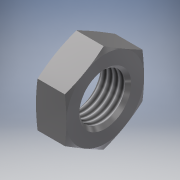
# Autodesk Inventor part: D-801
Saved by Autodesk Inventor 2016 SP2 (Build 200236200, 236)
## iProperties
Category: PARTsolutions
Company: BIMBA
Created: 2017-03-17
Part Number: D-801
Catalog Web Link: www.cadenas.de
Description: Jam Nut-Bimba Nut for Alignment Couplers
Vendor: BIMBA
Document SubType Name: Modeling
Designer: psAdmin
Manufacturer: BIMBA
Mass: 5.17328 g
Surface Area: 6.36956 cm^2
Volume: 0.659017 cm^3
Density: 7.85 g/cm^3
Material: Steel, Carbon
Appearance: Semi-Polished
PSOL_IDENT_0: {$CADENAS_DATA\23d-libs\bimba\bimba\bimba_imperial\bimba_full_line\related_products\ac_jam_nut.prj},
PSOL_IDENT_1: 156 {VTYP=3D},{NB=D-801},{LINA=D-801},{NN=Jam Nut},{DATE=01.09.2016 11:36:35},{GEOMDATE=06.09.2013 0
PSOL_IDENT_2: 7:06:46},{VERSION=},{LINEID=30},{LINESUBID=-1},{WBVAR=MAT}  {NB=D-801},{LINA=D-801},{KT=DUMMY},{PN=D
PSOL_IDENT_3: -801},{PN1=D-801},{SIZE=3/8-24},{MAT=},{J=0.22},{JJ=0.22000},{T=3/8-24},{TT=0.37500},{H=0.56},{HEX=0
PSOL_IDENT_4: .560},{COLOR=0.75,0.75,0.75,0.00}
NN: Jam Nut
NT: Bimba Nut for Alignment Couplers
NB: D-801
NBSYN: $PN.
LINA: D-801
PN: D-801
SIZE: 3/8-24 [D-801]
MAT: Zinc-Plated Carbon Steel
J: 0.22
T: 3/8-24
H: 0.56
SUPPLIER: BIMBA
ARTICLENO: D-801
BOMINFO: D-801
CREATOR: CADENAS GmbH
Title: D-801
Author: Cadenas PARTsolutions
Comments: Bimba Nut for Alignment Couplers
Autodesk Inventor part; units mm, degrees
sketch "Sketch_1" plane through (0, 0, 0) normal (0, 0, 1) x (1, 0, 0)
  line L0 (2.794, 0) -> (-2.794, 0)
  line L1 (-2.794, 4.7625) -> (-2.2212, 4.1897)
  line L2 (-2.2212, 4.1897) -> (2.2212, 4.1897)
  line L3 (2.2212, 4.1897) -> (2.794, 4.7625)
  line L4 (2.794, 4.7625) -> (2.794, 7.112)
  line L5 (2.794, 7.112) -> (2.4129, 8.5344)
  line L6 (2.4129, 8.5344) -> (-2.4129, 8.5344)
  line L7 (-2.4129, 8.5344) -> (-2.794, 7.112)
  line L8 (-2.794, 7.112) -> (-2.794, 4.7625)
  constraints: 18 end point
revolve "Revolution1" add sketch "Sketch_1" angle 360 about axis through (2.794, 0, 0) along (1, 0, 0)
thread "Thread1" size "3/8-24 UNF" class "2B" standard "ANSI Unified Screw Threads" full length
sketch "Sketch_2" plane through (0, 0, 0) normal (1, 0, 0) x (0, 1, 0)
  circle A0 centre (0, 0) radius 14.224
  line L0 (-4.1061, 7.112) -> (-8.2122, 0)
  line L1 (-8.2122, 0) -> (-4.1061, -7.112)
  line L2 (-4.1061, -7.112) -> (4.1061, -7.112)
  line L3 (4.1061, -7.112) -> (8.2122, 0)
  line L4 (8.2122, 0) -> (4.1061, 7.112)
  line L5 (4.1061, 7.112) -> (-4.1061, 7.112)
  constraints: 12 end point, 1 centre point
extrude "Extrusion1" cut sketch "Sketch_2" along normal mid plane 11.176
ref_plane "h1_XY" through (0, 0, 7.112) normal (1, 0, 0) x (0, 0, -1)
ref_plane "h1_YZ" through (0, 0, 7.112) normal (0, 0, -1) x (0, 1, 0)
ref_plane "h1_ZX" through (0, 0, 7.112) normal (0, 1, 0) x (1, 0, 0)
ref_plane "h2_XY" through (0, 0, -7.112) normal (1, 0, 0) x (0, 0, -1)
ref_plane "h2_YZ" through (0, 0, -7.112) normal (0, 0, -1) x (0, 1, 0)
ref_plane "h2_ZX" through (0, 0, -7.112) normal (0, 1, 0) x (1, 0, 0)
ref_plane "j1_XY" through (-2.794, 0, 0) normal (0, 0, 1) x (1, 0, 0)
ref_plane "j1_YZ" through (-2.794, 0, 0) normal (1, 0, 0) x (0, 1, 0)
ref_plane "j1_ZX" through (-2.794, 0, 0) normal (0, 1, 0) x (0, 0, 1)
ref_plane "j2_XY" through (2.794, 0, 0) normal (0, 0, 1) x (1, 0, 0)
ref_plane "j2_YZ" through (2.794, 0, 0) normal (1, 0, 0) x (0, 1, 0)
ref_plane "j2_ZX" through (2.794, 0, 0) normal (0, 1, 0) x (0, 0, 1)
ref_plane "jam_nut_XY" through (0, 0, 0) normal (1, 0, 0) x (0, 0, -1)
ref_plane "jam_nut_YZ" through (0, 0, 0) normal (0, 0, -1) x (0, 1, 0)
ref_plane "jam_nut_ZX" through (0, 0, 0) normal (0, 1, 0) x (1, 0, 0)
ref_plane "t1_XY" through (0, 0, 4.7625) normal (1, 0, 0) x (0, 0, -1)
ref_plane "t1_YZ" through (0, 0, 4.7625) normal (0, 0, -1) x (0, 1, 0)
ref_plane "t1_ZX" through (0, 0, 4.7625) normal (0, 1, 0) x (1, 0, 0)
ref_plane "t2_XY" through (0, 0, -4.7625) normal (1, 0, 0) x (0, 0, -1)
ref_plane "t2_YZ" through (0, 0, -4.7625) normal (0, 0, -1) x (0, 1, 0)
ref_plane "t2_ZX" through (0, 0, -4.7625) normal (0, 1, 0) x (1, 0, 0)
body "Solid1"
